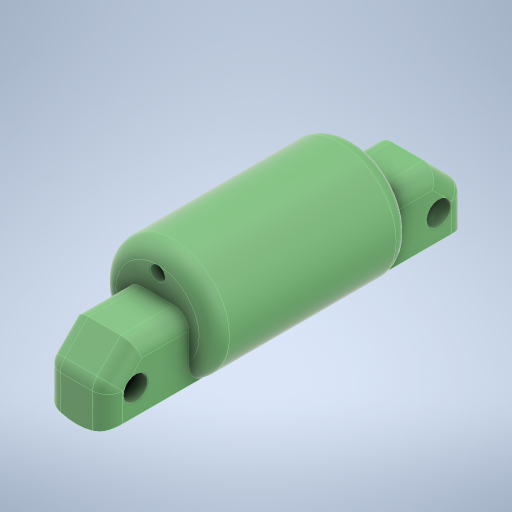
# Autodesk Inventor part: 零件2
Saved by Autodesk Inventor 2023 (Build 270158000, 158)
## iProperties
Created: 2023-09-13
Part Number: 零件2
Material: 常规
Document SubType Name: Modeling
Designer: Administrator
Density: 1 g/cm^3
Appearance: 平滑 - 深森林绿
Author: Administrator
Autodesk Inventor part; units mm, degrees
ref_plane "YZ Plane" through (0, 0, 0) normal (1, 0, 0) x (0, 1, 0)
ref_plane "XZ Plane" through (0, 0, 0) normal (0, 1, 0) x (-1, 0, 0)
ref_plane "XY Plane" through (0, 0, 0) normal (0, 0, 1) x (1, 0, 0)
sketch "草图1" plane through (0, 0, 0) normal (1, 0, 0) x (0, 1, 0)
  line L0 (0, 0) -> (7.5, 0)
  line L1 (7.5, 0) -> (7.5, -25)
  line L2 (7.5, -25) -> (0, -25)
  line L3 (0, -25) -> (0, 0)
  dimension "d0" = 25
  dimension "d1" = 7.5
  constraints: 8 end point, 2 parallel, 1 horizontal, 1 perpendicular
  measures "d0" distance of L0.end L1.end
  measures "d1" distance of L1.end L2.end
revolve "旋转1" add sketch "草图1" angle 360 about axis through (0, 0, -25) along (0, 0, 1)
sketch "草图2" plane through (0, 0, 0) normal (1, 0, 0) x (0, 1, 0)
  line L0 (12, -13) -> (2, -13)
  line L1 (2, -13) -> (2, -33)
  line L2 (2, -33) -> (12, -33)
  line L3 (12, -33) -> (12, -13)
  line L4 (7.5, -25) -> (-7.5, -25) projected
  point P0 (0, 0)
  point P1 (0, -25)
  dimension "d3" = 20
  dimension "d4" = 10
  dimension "d5" = 12
  dimension "d6" = 12
  constraints: 8 end point, 2 parallel, 1 horizontal, 1 midpoint, 1 perpendicular
  measures "d3" distance of L2.end L0.start
  measures "d4" distance of L1.end L2.end
  measures "d5" distance between parallel lines of L4 L0
  measures "d6" distance from line of point (0, -25) L3
extrude "拉伸1" cut sketch "草图2" along normal mid plane 20
sketch "草图3" plane through (0, 0, -25) normal (0, 0, 1) x (1, 0, 0)
  line L0 (8.125, 10) -> (4.125, 10)
  line L1 (4.125, 10) -> (4.125, -10)
  line L2 (4.125, -10) -> (8.125, -10)
  line L3 (8.125, -10) -> (8.125, 10)
  line L4 (-4.125, 10) -> (-8.125, 10)
  line L5 (-8.125, 10) -> (-8.125, -10)
  line L6 (-8.125, -10) -> (-4.125, -10)
  line L7 (-4.125, -10) -> (-4.125, 10)
  point P0 (0, 0)
  dimension "d9" = 4
  dimension "d10" = 20
  dimension "d11" = 10
  dimension "d12" = 8.125
  dimension "d13" = 4
  dimension "d14" = 4
  dimension "d15" = 20
  dimension "d16" = 4.125
  dimension "d17" = 10
  constraints: 16 end point, 4 parallel, 2 horizontal, 2 perpendicular
  measures "d9" distance of L0.start L0.end
  measures "d10" distance of L2.end L0.start
  measures "d11" distance from line of point (0, 0) L0
  measures "d12" distance from line of point (0, 0) L3
  measures "d13" distance of L1.end L2.end
  measures "d14" distance of L4.start L4.end
  measures "d15" distance of L4.end L5.end
  measures "d16" distance from line of point (0, 0) L7
  measures "d17" distance from line of point (0, 0) L6
extrude "拉伸2" cut sketch "草图3" along normal blind 12
sketch "草图6" plane through (0, 0, 0) normal (1, 0, 0) x (0, 1, 0)
  line L0 (2, -25) -> (-6.2637, -25) projected
  line L1 (2, -13) -> (2, -25) projected
  line L2 (2, -20) -> (-3, -25)
  point P0 (0, 0)
  dimension "d20" = 5
  dimension "d21" = 135
  constraints: 2 end point, 2 point on line
  measures "d20" horizontal distance of L2.start L2.end
  measures "d21" angle of L0 L2
extrude "拉伸3" cut sketch "草图6" along normal mid plane 100
sketch "草图7" plane through (0, 0, 0) normal (1, 0, 0) x (0, 1, 0)
  circle A0 centre (-3.0637, -20) radius 1.6
  line L0 (-6.2637, -13) -> (-6.2637, -25) projected
  line L1 (-6.2637, -25) -> (-3, -25) projected
  point P0 (0, 0)
  point P1 (-4.6319, -25)
  dimension "d24" = 3.2
  dimension "d25" = 3.2
  dimension "d26" = 5
  constraints: 1 centre point, 1 midpoint
  measures "d24" diameter of A0
  measures "d25" distance from line of A0.centre L0
  measures "d26" vertical distance of point (-4.632, -25) A0.centre
extrude "拉伸4" cut sketch "草图7" along normal mid plane 100
mirror "镜像1" about plane through (0, 0, 0) normal (0, 0, 1)
sketch "草图8" plane through (0, 0, 13) normal (0, 0, 1) x (1, 0, 0)
  circle A0 centre (0, 4.5) radius 1
  line L0 (4.125, 2) -> (-4.125, 2) projected
  point P0 (0, 0)
  dimension "d29" = 2
  dimension "d30" = 4.5
  dimension "d31" = 2.5
  constraints: 1 centre point
  measures "d29" diameter of A0
  measures "d30" distance of point (0, 0) A0.centre
  measures "d31" distance from line of L0 A0.centre
extrude "拉伸5" cut sketch "草图8" against normal blind 100
fillet "圆角1" radius 2 14 edges at (7.1843, 2.1531, -13) (-7.1843, 2.1531, -13) (7.1843, 2.1531, 13) (-7.1843, 2.1531, 13) (4.125, -0.5, -22.5) (4.125, 2, -16.5) (-4.125, 2, -16.5) (-4.125, -0.5, -22.5) (0, -7.5, -25) (4.125, -0.5, 22.5) (4.125, 2, 16.5) (-4.125, 2, 16.5) (-4.125, -0.5, 22.5) (0, -7.5, 25)
sketch "草图9" plane through (0, 0, 0) normal (1, 0, 0) x (0, 1, 0)
  line L0 (5.9687, -34.7753) -> (-21.5537, -34.7753)
  line L1 (-21.5537, -34.7753) -> (-21.5537, -23.7)
  line L2 (-21.5537, -23.7) -> (5.9687, -23.7)
  line L3 (5.9687, -23.7) -> (5.9687, -34.7753)
  line L4 (4.8413, 23.7) -> (-20.161, 23.7)
  line L5 (-20.161, 23.7) -> (-20.161, 41.0756)
  line L6 (-20.161, 41.0756) -> (4.8413, 41.0756)
  line L7 (4.8413, 41.0756) -> (4.8413, 23.7)
  line L8 (7.5, 11) -> (-6.2637, 11) projected
  line L9 (-6.2637, 11) -> (-6.2637, 23) projected
  line L10 (-6.2637, -11) -> (-6.2637, -23) projected
  line L11 (-6.2637, -11) -> (7.5, -11) projected
  point P0 (0, 0)
  dimension "d35" = 11.0753
  dimension "d36" = 27.5224
  dimension "d37" = 17.3756
  dimension "d38" = 25.0023
  dimension "d39" = 12.7
  dimension "d40" = 13.8972
  dimension "d41" = 12.2325
  dimension "d42" = 12.7
  constraints: 16 end point, 4 parallel, 2 horizontal, 2 perpendicular
  measures "d35" distance of L2.end L0.start
  measures "d36" distance of L0.start L0.end
  measures "d37" distance of L6.end L4.start
  measures "d38" distance of L5.end L6.end
  measures "d39" distance between parallel lines of L4 L8
  measures "d40" distance between parallel lines of L9 L5
  measures "d41" distance between parallel lines of L10 L3
  measures "d42" distance between parallel lines of L11 L2
extrude "拉伸6" cut sketch "草图9" along normal mid plane 100
fillet "圆角2" radius 2 5 edges at (-4.125, -5.3201, -23.7) (0, -1.7, -23.7) (3.5392, -2.5284, -23.7) (4.125, -5.3201, -23.7) (-3.5392, -2.5284, -23.7)
fillet "圆角3" radius 2 5 edges at (3.5392, -2.5284, 23.7) (4.125, -5.3201, 23.7) (-3.5392, -2.5284, 23.7) (-4.125, -5.3201, 23.7) (0, -1.7, 23.7)
